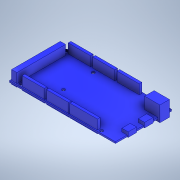
# Autodesk Inventor part: Carte Due
Saved by Autodesk Inventor 2020 (Build 240168000, 168)
## iProperties
Created: 2020-01-01
Part Number: Carte Due
Material: Argent
Document SubType Name: Modeling
Designer: Manuel Enzo
Density: 10.49 g/cm^3
Appearance: Bleu - Peinture murale - Brillant
Author: Manuel Enzo
Autodesk Inventor part; units mm, degrees
ref_plane "YZ Plane" through (0, 0, 0) normal (1, 0, 0) x (0, 1, 0)
ref_plane "XZ Plane" through (0, 0, 0) normal (0, 1, 0) x (-1, 0, 0)
ref_plane "XY Plane" through (0, 0, 0) normal (0, 0, 1) x (1, 0, 0)
sketch "Esquisse1" plane through (0, 0, 0) normal (0, 1, 0) x (-1, 0, 0)
  line L0 (0, 0) -> (100, 0)
  line L1 (100, 0) -> (100, -53)
  line L2 (100, -53) -> (0, -53)
  line L3 (0, -53) -> (0, 0)
  line L4 (100, -48) -> (103, -48)
  line L5 (103, -48) -> (103, -15)
  line L6 (103, -15) -> (100, -15)
  line L7 (100, -15) -> (100, -48)
  line L8 (103, -48) -> (100, -51)
  line L9 (103, -15) -> (100, -12)
  line L10 (99, -1) -> (94, -1)
  line L11 (94, -1) -> (94, -47)
  line L12 (94, -47) -> (99, -47)
  line L13 (99, -47) -> (99, -1)
  circle A0 centre (91.5, -2.5) radius 2.5
  circle A1 centre (91.5, -2.5) radius 1.5
  circle A2 centre (97.5, -50.5) radius 2.5
  circle A3 centre (97.5, -50.5) radius 1.5
  line L14 (89, -3.5) -> (68, -3.5)
  line L15 (68, -3.5) -> (68, -1)
  line L16 (68, -1) -> (89, -1)
  line L17 (89, -1) -> (89, -3.5)
  line L18 (66, -3.5) -> (45, -3.5)
  line L19 (45, -3.5) -> (45, -1)
  line L20 (45, -1) -> (66, -1)
  line L21 (66, -1) -> (66, -3.5)
  line L22 (44, -3.5) -> (18, -3.5)
  line L23 (18, -3.5) -> (18, -1)
  line L24 (18, -1) -> (44, -1)
  line L25 (44, -1) -> (44, -3.5)
  circle A4 centre (15.5, -2.5) radius 2.5
  circle A5 centre (15.5, -2.5) radius 1.5
  line L26 (94, -52) -> (73, -52)
  line L27 (73, -52) -> (73, -49.5)
  line L28 (73, -49.5) -> (94, -49.5)
  line L29 (94, -49.5) -> (94, -52)
  line L30 (71, -52) -> (50, -52)
  line L31 (50, -52) -> (50, -49.5)
  line L32 (50, -49.5) -> (71, -49.5)
  line L33 (71, -49.5) -> (71, -52)
  line L34 (48, -52) -> (27, -52)
  line L35 (27, -52) -> (27, -49.5)
  line L36 (27, -49.5) -> (48, -49.5)
  line L37 (48, -49.5) -> (48, -52)
  circle A6 centre (15.5, -50.5) radius 2.5
  circle A7 centre (15.5, -50.5) radius 1.5
  line L38 (5, -11) -> (-1, -11)
  line L39 (-1, -11) -> (-1, -19)
  line L40 (-1, -19) -> (5, -19)
  line L41 (5, -19) -> (5, -11)
  line L42 (5, -26.5) -> (-1, -26.5)
  line L43 (-1, -26.5) -> (-1, -34.5)
  line L44 (-1, -34.5) -> (5, -34.5)
  line L45 (5, -34.5) -> (5, -26.5)
  line L46 (12.5, -40) -> (-2, -40)
  line L47 (-2, -40) -> (-2, -49)
  line L48 (-2, -49) -> (12.5, -49)
  line L49 (12.5, -49) -> (12.5, -40)
  circle A8 centre (67, -18) radius 2.5
  circle A9 centre (67, -18) radius 1.5
  circle A10 centre (67, -46) radius 2.5
  circle A11 centre (67, -46) radius 1.5
  point P0 (0, -11)
  point P1 (0, -19)
  point P2 (0, -26.5)
  point P3 (0, -34.5)
  point P4 (0, -40)
  point P5 (0, -49)
  point P6 (97.5, -53)
  point P7 (100, -50.5)
  dimension "d0" = 53
  dimension "d1" = 100
  dimension "d2" = 3
  dimension "d3" = 5
  dimension "d4" = 15
  dimension "d5" = 45
  dimension "d6" = 45
  dimension "d7" = 1
  dimension "d8" = 1
  dimension "d9" = 5
  dimension "d10" = 46
  dimension "d11" = 1
  dimension "d12" = 5
  dimension "d13" = 2.5
  dimension "d14" = 2.5
  dimension "d15" = 1
  dimension "d16" = 5
  dimension "d17" = 2.5
  dimension "d18" = 2.5
  dimension "d19" = 1
  dimension "d20" = 2.5
  dimension "d21" = 21
  dimension "d22" = 2.5
  dimension "d23" = 1
  dimension "d24" = 2.5
  dimension "d25" = 21
  dimension "d26" = 2
  dimension "d27" = 1
  dimension "d28" = 26
  dimension "d29" = 1
  dimension "d30" = 2.5
  dimension "d31" = 1
  dimension "d32" = 5
  dimension "d33" = 0
  dimension "d34" = 2.5
  dimension "d35" = 1
  dimension "d36" = 2.5
  dimension "d37" = 6
  dimension "d38" = 21
  dimension "d39" = 21
  dimension "d40" = 2
  dimension "d41" = 2
  dimension "d42" = 21
  dimension "d43" = 1
  dimension "d44" = 1
  dimension "d45" = 2.5
  dimension "d46" = 2.5
  dimension "d47" = 1
  dimension "d48" = 5
  dimension "d49" = 2.5
  dimension "d50" = 2.5
  dimension "d51" = 8
  dimension "d52" = 11
  dimension "d53" = 6
  dimension "d54" = 1
  dimension "d55" = 7.5
  dimension "d56" = 1
  dimension "d57" = 6
  dimension "d58" = 8
  dimension "d59" = 5.5
  dimension "d60" = 9
  dimension "d61" = 14.5
  dimension "d62" = 2
  dimension "d63" = 1
  constraints: 100 end point, 24 parallel, 13 perpendicular, 12 centre point, 12 horizontal, 6 coincident, 5 point on line
  measures "d0" distance between parallel lines of L0 L2
  measures "d1" distance between parallel lines of L3 L1
  measures "d2" distance between parallel lines of L5 L1
  measures "d3" distance between parallel lines of L2 L4
  measures "d4" distance between parallel lines of L0 L6
  measures "d5" angle of L9 L6
  measures "d6" angle of L4 L8
  measures "d7" distance between parallel lines of L7 L13
  measures "d8" distance between parallel lines of L0 L10
  measures "d9" distance between parallel lines of L13 L11
  measures "d10" distance between parallel lines of L12 L10
  measures "d11" radial gap between concentric circles of A0 A1
  measures "d12" diameter of A0
  measures "d13" distance from line of L11 A0.centre
  measures "d14" distance from line of L0 A0.centre
  measures "d15" radial gap between concentric circles of A2 A3
  measures "d16" diameter of A2
  measures "d17" distance from line of L1 A2.centre
  measures "d18" distance from line of L2 A3.centre
  measures "d19" distance between parallel lines of L0 L16
  measures "d20" distance between parallel lines of L16 L14
  measures "d21" distance between parallel lines of L15 L17
  measures "d22" distance from line of L17 A0.centre
  measures "d23" distance between parallel lines of L0 L20
  measures "d24" distance between parallel lines of L20 L18
  measures "d25" distance between parallel lines of L21 L19
  measures "d26" distance between parallel lines of L15 L21
  measures "d27" distance from line of L19 L24.end
  measures "d28" distance between parallel lines of L25 L23
  measures "d29" distance between parallel lines of L0 L24
  measures "d30" distance between parallel lines of L24 L22
  measures "d31" radial gap between concentric circles of A4 A5
  measures "d32" diameter of A4
  measures "d33" distance edge to line of A4 L23
  measures "d34" distance from line of L0 A4.centre
  measures "d35" distance between parallel lines of L2 L26
  measures "d36" distance between parallel lines of L26 L28
  measures "d37" distance from line of L7 L26.start
  measures "d38" distance between parallel lines of L27 L29
  measures "d39" distance between parallel lines of L31 L33
  measures "d40" distance between parallel lines of L27 L33
  measures "d41" distance between parallel lines of L37 L31
  measures "d42" distance from line of L37 L35.end
  measures "d43" distance between parallel lines of L2 L34
  measures "d44" distance between parallel lines of L2 L30
  measures "d45" distance between parallel lines of L30 L32
  measures "d46" distance between parallel lines of L34 L36
  measures "d47" radial gap between concentric circles of A6 A7
  measures "d48" diameter of A6
  measures "d49" distance from line of L2 A7.centre
  measures "d50" distance from line of A6.centre L23
  measures "d51" distance between parallel lines of L38 L40
  measures "d52" distance between parallel lines of L0 L38
  measures "d53" distance between parallel lines of L39 L41
  measures "d54" distance between parallel lines of L3 L39
  measures "d55" distance between parallel lines of L40 L42
  measures "d56" distance between parallel lines of L3 L43
  measures "d57" distance between parallel lines of L43 L45
  measures "d58" distance between parallel lines of L42 L44
  measures "d59" distance between parallel lines of L46 L44
  measures "d60" distance between parallel lines of L46 L48
  measures "d61" distance between parallel lines of L49 L47
  measures "d62" distance between parallel lines of L3 L47
  measures "d63" radial gap between concentric circles of A8 A9
extrude "Extrusion1" add sketch "Esquisse1" along normal blind 1.5 contours A6 | A0 | A4 | L0 L1 A2 L2 L3 L48 L49 L46 L44 L45 L42 L40 L41 L38 | L9 L6 L1 | L6 L5 L4 L1 | L4 L8 L1 | A2 | A1 | A8 | A10
extrude "Extrusion2" cut sketch "Esquisse1" along normal through all contours A1
extrude "Extrusion3" add sketch "Esquisse1" along normal blind 10.5 contours L11 L10 L13 L12 | L17 L14 L15 L16 | L23 L24 L25 L22 | L18 L19 L20 L21 | L26 L27 L28 L29 | L30 L31 L32 L33 | L34 L35 L36 L37
extrude "Extrusion4" add sketch "Esquisse1" along normal blind 4.5 contours L38 L41 L40 L3 | L3 L40 L39 L38 | L42 L45 L44 L3 | L3 L44 L43 L42
extrude "Extrusion5" add sketch "Esquisse1" along normal blind 12.5 contours L46 L49 L48 L3 | L3 L48 L47 L46
extrude "Extrusion6" add sketch "Esquisse1" against normal blind 1.5 contours L11 L10 L13 L12 | L17 L14 L15 L16 | L23 L24 L25 L22 | L18 L19 L20 L21 | L26 L27 L28 L29 | L30 L31 L32 L33 | L34 L35 L36 L37
extrude "Extrusion7" add sketch "Esquisse1" against normal blind 2 contours L46 L49 L48 L3 | L3 L48 L47 L46
